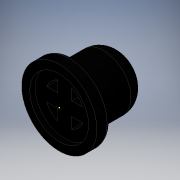
# Autodesk Inventor part: Button
Saved by Autodesk Inventor 2016 SP1 (Build 200210100, 210)
## iProperties
Created: 2018-06-05
Part Number: Button
Material: Plastique ABS
Document SubType Name: Modeling
Designer: dimercur
Density: 1.06 g/cm^3
Appearance: Noir
Author: dimercur
Autodesk Inventor part; units mm, degrees
ref_plane "YZ Plane" through (0, 0, 0) normal (1, 0, 0) x (0, 1, 0)
ref_plane "XZ Plane" through (0, 0, 0) normal (0, 1, 0) x (-1, 0, 0)
ref_plane "XY Plane" through (0, 0, 0) normal (0, 0, 1) x (1, 0, 0)
sketch "Esquisse1" plane through (0, 0, 0) normal (0, 1, 0) x (-1, 0, 0)
  circle A0 centre (0, 0) radius 4
  dimension "d0" = 8
  constraints: 1 centre point, 1 coincident
  measures "d0" diameter of A0
extrude "Extrusion1" add sketch "Esquisse1" along normal blind 7
fillet "Congé1" radius 2.5 1 edges at (4, 7, 0)
sketch "Esquisse2" plane through (0, 0, 0) normal (0, -1, 0) x (1, 0, 0)
  circle A0 centre (0, 0) radius 5.5
  dimension "d4" = 11
  constraints: 1 centre point, 1 coincident
  measures "d4" diameter of A0
extrude "Extrusion2" add sketch "Esquisse2" along normal blind 2
sketch "Esquisse3" plane through (0, -2, 0) normal (0, -1, 0) x (1, 0, 0)
  point P0 (0, 0)
shell "Coque1" thickness 1.2 removed faces 1 at (1.6766, -2, 0.4132)
sketch "Esquisse4" plane through (0, -1.2, 0) normal (0, -1, 0) x (1, 0, 0)
  line L0 (3.5, 1) -> (-3.5, 1)
  line L1 (-3.5, 1) -> (-3.5, -1)
  line L2 (-3.5, -1) -> (3.5, -1)
  line L3 (3.5, -1) -> (3.5, 1)
  line L4 (1, 3.5) -> (-1, 3.5)
  line L5 (-1, 3.5) -> (-1, -3.5)
  line L6 (-1, -3.5) -> (1, -3.5)
  line L7 (1, -3.5) -> (1, 3.5)
  point P0 (0, 0)
  dimension "d8" = 2
  dimension "d9" = 2
  dimension "d10" = 7
  dimension "d11" = 3.5
  dimension "d12" = 7
  dimension "d13" = 3.5
  dimension "d14" = 1
  dimension "d15" = 1
  constraints: 16 end point, 4 parallel, 2 horizontal, 2 perpendicular
  measures "d8" distance of L2.end L0.start
  measures "d9" distance of L4.start L4.end
  measures "d10" distance of L1.end L2.end
  measures "d11" horizontal distance of point (0, 0) L2.end
  measures "d12" distance of L6.end L4.start
  measures "d13" vertical distance of point (0, 0) L4.start
  measures "d14" horizontal distance of point (0, 0) L6.end
  measures "d15" vertical distance of point (0, 0) L0.start
extrude "Extrusion3" add sketch "Esquisse4" against normal blind 2
fillet "Congé2" radius 0.5 1 edges at (-5.5, 0, 0)
equation "\"d9\" = d8"
equation "\"d11\" = 0.5 * d10"
equation "\"d12\" = d10"
equation "\"d13\" = 0.5 * d12"
equation "\"d14\" = 0.5 * d9"
equation "\"d15\" = 0.5 * d8"
